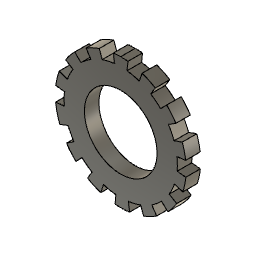
ATC 3D Drawing 7 v0 (Autodesk Fusion 360 design; units mm, degrees)
Autodesk Fusion 360 part; units mm, degrees
sketch "Sketch1" plane through (0, 0, 0) normal (0, 1, 0) x (1, 0, 0)
  circle A0 centre (0, 0) radius 25
  line L0 (0, 0) -> (0, -72.8192) construction
  line L1 (0, -72.8192) -> (0, 0) construction
  line L2 (0, -45) -> (-4.9923, -44.7222)
  line L3 (-4.9923, -44.7222) -> (-4.3266, -38.7593)
  line L4 (-14.7457, -42.5154) -> (-12.7796, -36.8467)
  line L5 (-23.771, -38.2091) -> (-20.6016, -33.1146)
  line L6 (-31.6224, -32.016) -> (-27.4061, -27.7472)
  line L7 (-37.9122, -24.2417) -> (-32.8573, -21.0095)
  line L8 (-42.3298, -15.2704) -> (-36.6859, -13.2344)
  line L9 (-44.6571, -5.545) -> (-38.7028, -4.8057)
  line L10 (0, 0) -> (-2.7735, -24.8457) construction
  line L11 (-4.3266, -38.7593) -> (-4.9923, -44.7222) construction
  line L12 (0, 0) -> (-8.1921, -23.6197) construction
  line L13 (-12.7796, -36.8467) -> (-14.7457, -42.5154) construction
  line L14 (0, 0) -> (-13.2061, -21.2273) construction
  line L15 (-20.6016, -33.1146) -> (-23.771, -38.2091) construction
  line L16 (0, 0) -> (-17.568, -17.7866) construction
  line L17 (-27.4061, -27.7472) -> (-31.6224, -32.016) construction
  line L18 (0, 0) -> (-21.0624, -13.4676) construction
  line L19 (-32.8573, -21.0095) -> (-37.9122, -24.2417) construction
  line L20 (0, 0) -> (-23.5166, -8.4836) construction
  line L21 (-36.6859, -13.2344) -> (-42.3298, -15.2704) construction
  line L22 (0, 0) -> (-24.8095, -3.0805) construction
  line L23 (-38.7028, -4.8057) -> (-44.6571, -5.545) construction
  arc A1 (-23.771, -38.2091) -> (-14.7457, -42.5154) centre (0, 0) ccw
  arc A2 (-37.9122, -24.2417) -> (-31.6224, -32.016) centre (0, 0) ccw
  arc A3 (-36.6859, -13.2344) -> (-32.8573, -21.0095) centre (0, 0) ccw
  arc A4 (-27.4061, -27.7472) -> (-20.6016, -33.1146) centre (0, 0) ccw
  line L24 (-44.7805, 4.4388) -> (-38.8098, 3.847) construction
  line L25 (0, 0) -> (-24.8781, 2.466) construction
  line L26 (-38.8098, 3.847) -> (-44.7805, 4.4388) construction
  line L27 (-44.7805, 4.4388) -> (-38.8098, 3.847)
  arc A5 (-44.6571, -5.545) -> (-42.3298, -15.2704) centre (0, 0) ccw
  line L28 (0, -45) -> (4.9923, -44.7222)
  line L29 (0, 0) -> (4.9923, -44.7222) construction
  line L30 (4.9923, -44.7222) -> (4.3266, -38.7593)
  line L31 (0.0235, -39) -> (0, -45) construction
  line L32 (0.0235, -39) -> (0, -45)
  arc A6 (-12.7796, -36.8467) -> (-4.3266, -38.7593) centre (0, 0) ccw
  line L33 (0, 0) -> (67, 0) construction
  line L34 (0, 0) -> (0, 30) construction
  line L35 (65.5098, -16.7592) -> (65.5098, -18.6386)
  line L36 (0, 0) -> (14.7457, -42.5154) construction
  line L37 (0, 0) -> (23.771, -38.2091) construction
  line L38 (0, 0) -> (31.6224, -32.016) construction
  line L39 (0, 0) -> (37.9122, -24.2417) construction
  line L40 (0, 0) -> (42.3298, -15.2704) construction
  line L41 (0, 0) -> (44.6571, -5.545) construction
  line L42 (12.7796, -36.8467) -> (14.7457, -42.5154)
  line L43 (20.6016, -33.1146) -> (23.771, -38.2091)
  line L44 (27.4061, -27.7472) -> (31.6224, -32.016)
  line L45 (32.8573, -21.0095) -> (37.9122, -24.2417)
  line L46 (36.6859, -13.2344) -> (42.3298, -15.2704)
  line L47 (38.7028, -4.8057) -> (44.6571, -5.545)
  arc A7 (-4.9923, -44.7222) -> (4.9923, -44.7222) centre (0, 0) ccw
  line L48 (4.9923, -44.7222) -> (14.7457, -42.5154) construction
  arc A8 (14.7457, -42.5154) -> (23.771, -38.2091) centre (0, 0) ccw
  line L49 (23.771, -38.2091) -> (31.6224, -32.016) construction
  arc A9 (31.6224, -32.016) -> (37.9122, -24.2417) centre (0, 0) ccw
  line L50 (37.9122, -24.2417) -> (42.3298, -15.2704) construction
  arc A10 (4.3266, -38.7593) -> (12.7796, -36.8467) centre (0, 0) ccw
  line L51 (12.7796, -36.8467) -> (20.6016, -33.1146) construction
  arc A11 (20.6016, -33.1146) -> (27.4061, -27.7472) centre (0, 0) ccw
  line L52 (27.4061, -27.7472) -> (32.8573, -21.0095) construction
  arc A12 (32.8573, -21.0095) -> (36.6859, -13.2344) centre (0, 0) ccw
  line L53 (36.6859, -13.2344) -> (38.7028, -4.8057) construction
  line L54 (-38.7028, -4.8057) -> (-36.6859, -13.2344) construction
  line L55 (-32.8573, -21.0095) -> (-27.4061, -27.7472) construction
  line L56 (-20.6016, -33.1146) -> (-12.7796, -36.8467) construction
  line L57 (-4.3266, -38.7593) -> (4.3266, -38.7593) construction
  line L58 (44.9966, -0.5565) -> (44.9725, 0)
  line L59 (0, 0) -> (44.7805, 4.4388) construction
  line L60 (0, 0) -> (42.6946, 14.2188) construction
  line L61 (0, 0) -> (38.5002, 23.2967) construction
  line L62 (0, 0) -> (32.4046, 31.2241) construction
  line L63 (0, 0) -> (24.7088, 37.6095) construction
  line L64 (0, 0) -> (15.7927, 42.1377) construction
  line L65 (0, 0) -> (6.0968, 44.5851) construction
  line L66 (38.8098, 3.847) -> (44.7805, 4.4388)
  line L67 (37.0019, 12.323) -> (42.6946, 14.2188)
  line L68 (33.3668, 20.1904) -> (38.5002, 23.2967)
  line L69 (28.084, 27.0609) -> (32.4046, 31.2241)
  line L70 (21.4143, 32.5949) -> (24.7088, 37.6095)
  line L71 (13.687, 36.5194) -> (15.7927, 42.1377)
  line L72 (5.2839, 38.6404) -> (6.0968, 44.5851)
  arc A13 (42.3298, -15.2704) -> (44.6571, -5.545) centre (0, 0) ccw
  arc A14 (44.9966, -0.5565) -> (45, 0) centre (0, 0) ccw
  line L73 (44.6571, -5.545) -> (44.7805, 4.4388) construction
  arc A15 (44.7805, 4.4388) -> (42.6946, 14.2188) centre (0, 0) ccw
  line L74 (42.6946, 14.2188) -> (38.5002, 23.2967) construction
  arc A16 (38.5002, 23.2967) -> (32.4046, 31.2241) centre (0, 0) ccw
  line L75 (32.4046, 31.2241) -> (24.7088, 37.6095) construction
  arc A17 (24.7088, 37.6095) -> (15.7927, 42.1377) centre (0, 0) ccw
  line L76 (15.7927, 42.1377) -> (6.0968, 44.5851) construction
  line L77 (1.113, 44.9862) -> (-3.8847, 44.832)
  line L78 (0, 0) -> (-3.8847, 44.832) construction
  line L79 (0, 0) -> (-13.6897, 42.8671) construction
  line L80 (0, 0) -> (-22.8188, 38.7854) construction
  line L81 (0, 0) -> (-30.8209, 32.7883) construction
  line L82 (0, 0) -> (-37.3011, 25.172) construction
  line L83 (0, 0) -> (-41.9392, 16.3127) construction
  line L84 (-3.3667, 38.8544) -> (-3.8847, 44.832)
  line L85 (-11.8644, 37.1515) -> (-13.6897, 42.8671)
  line L86 (-19.7763, 33.614) -> (-22.8188, 38.7854)
  line L87 (-26.7115, 28.4165) -> (-30.8209, 32.7883)
  line L88 (-32.3276, 21.8157) -> (-37.3011, 25.172)
  line L89 (-41.9392, 16.3127) -> (-36.3473, 14.1376)
  arc A18 (6.0968, 44.5851) -> (-3.8847, 44.832) centre (0, 0) ccw
  line L90 (-3.8847, 44.832) -> (-13.6897, 42.8671) construction
  line L91 (-13.6897, 42.8671) -> (-11.8644, 37.1515) construction
  arc A19 (-13.6897, 42.8671) -> (-22.8188, 38.7854) centre (0, 0) ccw
  line L92 (-22.8188, 38.7854) -> (-30.8209, 32.7883) construction
  line L93 (-30.8209, 32.7883) -> (-26.7115, 28.4165) construction
  line L94 (-30.8209, 32.7883) -> (-26.7115, 28.4165)
  arc A20 (-30.8209, 32.7883) -> (-37.3011, 25.172) centre (0, 0) ccw
  arc A21 (-41.9392, 16.3127) -> (-44.7805, 4.4388) centre (0, 0) ccw
  line L95 (-37.3011, 25.172) -> (-41.9392, 16.3127) construction
  line L96 (-41.9392, 16.3127) -> (-36.3473, 14.1376)
  line L97 (-32.3276, 21.8157) -> (-37.3011, 25.172)
  arc A22 (38.7028, -4.8057) -> (38.8098, 3.847) centre (0, 0) ccw
  line L98 (38.8098, 3.847) -> (37.0019, 12.323) construction
  line L99 (24.7088, 37.6095) -> (21.4143, 32.5949)
  arc A23 (37.0019, 12.323) -> (33.3668, 20.1904) centre (0, 0) ccw
  line L100 (33.3668, 20.1904) -> (28.084, 27.0609) construction
  line L101 (38.5002, 23.2967) -> (33.3668, 20.1904)
  arc A24 (28.084, 27.0609) -> (21.4143, 32.5949) centre (0, 0) ccw
  line L102 (21.4143, 32.5949) -> (13.687, 36.5194) construction
  line L103 (13.687, 36.5194) -> (15.7927, 42.1377)
  arc A25 (13.687, 36.5194) -> (5.2839, 38.6404) centre (0, 0) ccw
  line L104 (5.2839, 38.6404) -> (-3.3667, 38.8544) construction
  line L105 (-3.3667, 38.8544) -> (-3.8847, 44.832)
  line L106 (-13.6897, 42.8671) -> (-11.8644, 37.1515)
  arc A26 (-3.3667, 38.8544) -> (-11.8644, 37.1515) centre (0, 0) ccw
  line L107 (-11.8644, 37.1515) -> (-19.7763, 33.614) construction
  line L108 (-22.8188, 38.7854) -> (-19.7763, 33.614)
  line L109 (-30.8209, 32.7883) -> (-26.7115, 28.4165)
  arc A27 (-19.7763, 33.614) -> (-26.7115, 28.4165) centre (0, 0) ccw
  line L110 (-26.7115, 28.4165) -> (-32.3276, 21.8157) construction
  line L111 (-37.3011, 25.172) -> (-32.3276, 21.8157)
  line L112 (-36.3473, 14.1376) -> (-41.9392, 16.3127)
  arc A28 (-32.3276, 21.8157) -> (-36.3473, 14.1376) centre (0, 0) ccw
  arc A29 (-38.8098, 3.847) -> (-38.7028, -4.8057) centre (0, 0) ccw
  line L113 (-38.8098, 3.847) -> (-36.3473, 14.1376) construction
  line L114 (-41.9392, 16.3127) -> (-36.3473, 14.1376)
  line L115 (-32.3276, 21.8157) -> (-36.3473, 14.1376)
  dimension "d1" = 90
  dimension "d2" = 78
  dimension "d3" = 50
  dimension "d4" = 5
  dimension "d5" = 10
  dimension "d6" = 10
  dimension "d7" = 10
  dimension "d8" = 10
  dimension "d9" = 10
  dimension "d10" = 10
  dimension "d13" = 12.739
  dimension "d14" = 5
  dimension "d15" = 10
  dimension "d16" = 10
  dimension "d17" = 10
  dimension "d18" = 10
  dimension "d19" = 10
  dimension "d20" = 10
  dimension "d21" = 5
  dimension "d22" = 5
  dimension "d23" = 10
  dimension "d24" = 10
  dimension "d25" = 10
  dimension "d26" = 10
  dimension "d27" = 10
  dimension "d28" = 10
  dimension "d29" = 5
  dimension "d30" = 5
  dimension "d31" = 10
  dimension "d32" = 10
  dimension "d33" = 10
  dimension "d34" = 10
  dimension "d35" = 10
  constraint coincident A0.centre L0.start
  constraint concentric A3 A7
  constraint concentric A0 A7
  constraint vertical L0
  constraint coincident L2.start A7
  constraint coincident L1 L2.start
  constraint coincident L5.start A7
  constraint coincident L7.start A7
  constraint coincident L9.start A7
  constraint coincident L3.end A3
  constraint coincident L3.end L10
  constraint coincident L4.end A3
  constraint coincident L4.end L12
  constraint coincident L5.end A3
  constraint coincident L5.end L14
  constraint coincident L6.end L16
  constraint coincident L6.end A3
  constraint coincident L7.end L18
  constraint coincident L8.end L20
  constraint coincident L9.end L22
  constraint coincident A0 L10.end
  constraint collinear L10 L11
  constraint coincident A0 L12.end
  constraint collinear L12 L13
  constraint coincident A0 L14.end
  constraint collinear L14 L15
  constraint coincident A0 L16.end
  constraint collinear L16 L17
  constraint coincident A0 L18.end
  constraint collinear L18 L19
  constraint coincident A0 L20.end
  constraint collinear L20 L21
  constraint coincident A0 L22.end
  constraint collinear L22 L23
  constraint concentric A1 A7
  constraint concentric A2 A7
  constraint concentric A3 A4
  constraint concentric A4 A6
  constraint coincident L24.end L25
  constraint coincident L24.end A6
  constraint coincident A0 L25.end
  constraint collinear L25 L26
  constraint parallel L26 L27
  constraint concentric A5 A7
  constraint coincident L30.end A6
  constraint coincident L29 L30.end
  constraint coincident L31.start A6
  constraint parallel L31 L32
  constraint concentric A6 A10
  constraint horizontal L33
  constraint vertical L34
  constraint vertical L35
  constraint coincident L36.end A7
  constraint coincident L37.end A7
  constraint coincident L38.end A7
  constraint coincident L39.end A7
  constraint coincident L40.end A7
  constraint coincident L41.end A7
  constraint coincident L58.start A7
  constraint coincident L36 L42.start
  constraint coincident L43.start A10
  constraint coincident L37 L43.start
  constraint coincident L44.start A10
  constraint coincident L38 L44.start
  constraint coincident L45.start A10
  constraint coincident L39 L45.start
  constraint coincident L40 L46.start
  constraint coincident L46.start A10
  constraint coincident L41 L47.start
  constraint coincident L47.start A10
  constraint concentric A7 A8
  constraint concentric A8 A9
  constraint concentric A9 A13
  constraint concentric A10 A11
  constraint concentric A11 A12
  constraint concentric A12 A22
  constraint coincident L59.end A13
  constraint coincident L60.end A13
  constraint coincident L61.end A13
  constraint coincident L62.end A13
  constraint coincident L63.end A13
  constraint coincident L64.end A13
  constraint coincident L65.end A13
  constraint coincident L77.start A13
  constraint coincident L59 L66.start
  constraint coincident L60 L67.start
  constraint coincident L67.start A22
  constraint coincident L68.start A22
  constraint coincident L61 L68.start
  constraint coincident L62 L69.start
  constraint coincident L69.start A22
  constraint coincident L63 L70.start
  constraint coincident L70.start A22
  constraint coincident L64 L71.start
  constraint coincident L71.start A22
  constraint coincident L65 L72.start
  constraint coincident L72.start A22
  constraint concentric A13 A14
  constraint coincident L33 L58.end
  constraint coincident L33 A14.end
  constraint concentric A14 A15
  constraint concentric A15 A16
  constraint concentric A16 A17
  constraint concentric A17 A18
  constraint coincident L79.end A18
  constraint coincident L80.end A18
  constraint coincident L81.end A18
  constraint coincident L82.end A18
  constraint coincident L83.end A18
  constraint coincident L78 L84.start
  constraint coincident L84.start A22
  constraint coincident L85.start A22
  constraint coincident L79 L85.start
  constraint coincident L86.start A22
  constraint coincident L80 L86.start
  constraint coincident L87.start A22
  constraint coincident L81 L87.start
  constraint coincident L88.start A22
  constraint coincident L82 L88.start
  constraint coincident L89.end A22
  constraint coincident L83 L89.end
  constraint concentric A18 A19
  constraint parallel L85 L91
  constraint concentric A19 A20
  constraint parallel L87 L93
  constraint parallel L93 L94
  constraint concentric A20 A21
  constraint parallel L89 L96
  constraint parallel L88 L97
  constraint concentric A22 A23
  constraint parallel L70 L99
  constraint concentric A23 A24
  constraint parallel L68 L101
  constraint concentric A24 A25
  constraint parallel L71 L103
  constraint concentric A25 A26
  constraint parallel L84 L105
  constraint parallel L85 L106
  constraint concentric A26 A27
  constraint parallel L86 L108
  constraint parallel L87 L109
  constraint concentric A27 A28
  constraint parallel L97 L111
  constraint parallel L96 L112
  constraint concentric A28 A29
  constraint parallel L89 L114
  measures "d1" diameter of A7
  measures "d2" diameter of A3
  measures "d3" diameter of A0
  measures "d4" distance of L2.start L2.end
  measures "d5" distance of L2.end L4.start
  measures "d6" distance of L4.start L5.start
  measures "d7" distance of L5.start L6.start
  measures "d8" distance of L6.start L7.start
  measures "d9" distance of L7.start L8.start
  measures "d10" distance of L8.start L9.start
  measures "d13" angle of L23 L24
  measures "d14" distance of L2.start L28.end
  measures "d15" distance of L28.end L36.end
  measures "d16" distance of L36.end L37.end
  measures "d17" distance of L37.end L38.end
  measures "d18" distance of L38.end L39.end
  measures "d19" distance of L39.end L40.end
  measures "d20" distance of L40.end L41.end
  measures "d21" distance of L41.end L58.start
  measures "d22" distance of L58.start L59.end
  measures "d23" distance of L59.end L60.end
  measures "d24" distance of L60.end L61.end
  measures "d25" distance of L61.end L62.end
  measures "d26" distance of L62.end L63.end
  measures "d27" distance of L63.end L64.end
  measures "d28" distance of L64.end L65.end
  measures "d29" distance of L65.end L77.start
  measures "d30" distance of L77.start L77.end
  measures "d31" distance of L77.end L79.end
  measures "d32" distance of L79.end L80.end
  measures "d33" distance of L80.end L81.end
  measures "d34" distance of L81.end L82.end
  measures "d35" distance of L82.end L83.end
extrude "Extrude1" add sketch "Sketch1" along normal mid plane 10 contours L2 L3 L4 L5 L6 L7 L8 L9 A1 A2 A3 A4 L27 A5 L28 L30 A6 L42 L43 L44 L45 L46 L47 A8 A9 A10 A11 A12 L66 L67 L68 L69 L70 L71 L72 A13 A15 A16 A17 L77 L84 L85 L86 L87 L88 L89 A18 A19 L94 A20 A21 L96 L97 A22 L99 A23 L101 A24 L103 A25 L105 L106 A26 L108 L109 A27 L111 L112 A29 L114 L115
